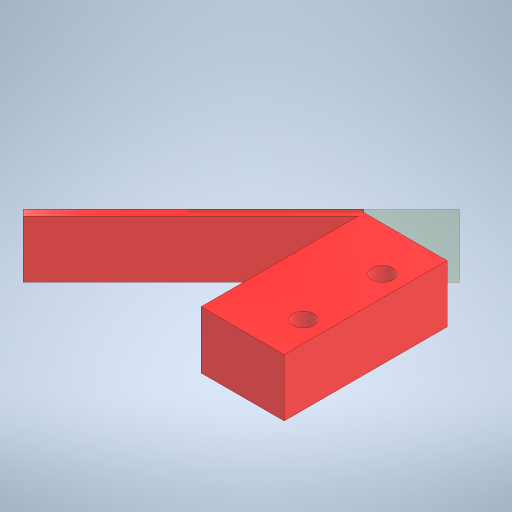
# Autodesk Inventor part: концевик
Saved by Autodesk Inventor 2023.1 (Build 271208000, 208)
## iProperties
Created: 2025-12-29
Part Number: концевик
Material: Типовые
Document SubType Name: Modeling
Designer: DELL
Density: 1 g/cm^3
Appearance: Светло-красный
Author: DELL
Autodesk Inventor part; units mm, degrees
ref_plane "YZ Plane" through (0, 0, 0) normal (1, 0, 0) x (0, 1, 0)
ref_plane "XZ Plane" through (0, 0, 0) normal (0, 1, 0) x (-1, 0, 0)
ref_plane "XY Plane" through (0, 0, 0) normal (0, 0, 1) x (1, 0, 0)
sketch "Эскиз1" plane through (0, 0, 0) normal (0, 1, 0) x (-1, 0, 0)
  line L0 (5, -9.8) -> (-5, -9.8)
  line L1 (-5, -9.8) -> (-5, 9.8)
  line L2 (-5, 9.8) -> (5, 9.8)
  line L3 (5, 9.8) -> (5, -9.8)
  line L4 (5, -9.8) -> (-5, 9.8) construction
  line L5 (-5, -9.8) -> (5, 9.8) construction
  point P0 (0, 0)
  dimension "d0" = 10
  dimension "d1" = 19.6
  constraints: 12 end point, 2 midpoint, 2 parallel, 1 horizontal, 1 perpendicular
  measures "d0" distance of L0.start L0.end
  measures "d1" distance of L0.end L1.end
extrude "Выдавливание1" add sketch "Эскиз1" along normal blind 6.9
sketch "Эскиз2" plane through (0, 6.9, 0) normal (0, 1, 0) x (1, 0, 0)
  circle A0 centre (2.5, -4.9766) radius 1.25
  circle A1 centre (2.5, 4.5234) radius 1.25
  line L0 (5, -9.8) -> (5, 9.8) projected
  line L1 (2.5, -4.9766) -> (2.5, -0.2266)
  line L2 (2.5, -0.2266) -> (2.5, 4.5234)
  point P0 (0, 0)
  dimension "d4" = 2.5
  dimension "d5" = 2.5
  dimension "d6" = 9.5
  dimension "d7" = 2.5
  dimension "d8" = 2.5
  constraints: 4 end point, 2 centre point, 1 collinear, 1 vertical
  measures "d4" diameter of A0
  measures "d5" diameter of A1
  measures "d6" distance of L1.start L2.end
  measures "d7" distance from line of L0 L1.start
  measures "d8" distance from line of L0 L2.end
extrude "Выдавливание2" cut sketch "Эскиз2" against normal blind 6.9
ref_plane "РабПлоскость1" through (-5, 0, -9.8) normal (-0.7071068, 0, -0.7071068) x (0, 1, 0)
sketch "Эскиз3" plane through (-5, 0, -9.8) normal (-0.7071068, 0, -0.7071068) x (0, 1, 0)
  line L0 (0, 0) -> (6.9, 0) projected
  line L1 (0, 0) -> (6.9, 0)
  line L2 (6.9, 0) -> (6.9, -29)
  line L3 (6.9, -29) -> (0, -29)
  line L4 (0, -29) -> (0, 0)
  point P0 (0, -3.3941)
  dimension "d12" = 6.9
  dimension "d13" = 29
  constraints: 8 end point, 2 parallel, 1 horizontal, 1 perpendicular
  measures "d12" distance of L2.end L3.end
  measures "d13" distance of L1.end L2.end
extrude "Выдавливание3" add sketch "Эскиз3" along normal mid plane 1
